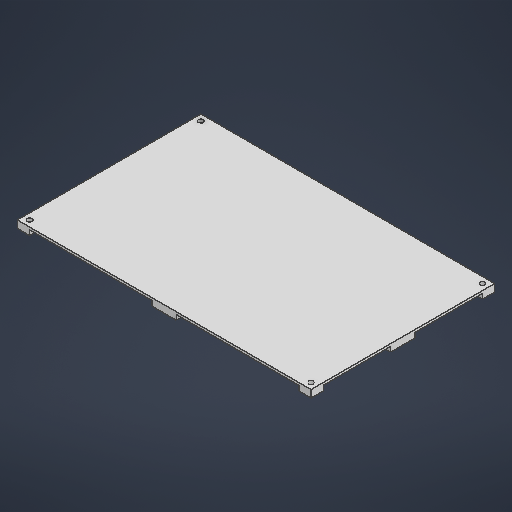
# Autodesk Inventor part: yellow_plate_cover
Saved by Autodesk Inventor 2026.1 (Build 301233000, 233)
## iProperties
Created: 2025-10-15
Part Number: yellow_plate_cover
Material: Generic
Document SubType Name: Modeling
Designer: emanuel
Density: 1 g/cm^3
Appearance: Default
Author: emanuel
Autodesk Inventor part; units mm, degrees
ref_plane "YZ Plane" through (0, 0, 0) normal (1, 0, 0) x (0, 1, 0)
ref_plane "XZ Plane" through (0, 0, 0) normal (0, 1, 0) x (-1, 0, 0)
ref_plane "XY Plane" through (0, 0, 0) normal (0, 0, 1) x (1, 0, 0)
sketch "Sketch1" plane through (0, 0, 0) normal (0, 1, 0) x (-1, 0, 0)
  line L0 (0, 0) -> (120, 0)
  line L1 (120, 0) -> (120, -75)
  line L2 (120, -75) -> (0, -75)
  line L3 (0, -75) -> (0, 0)
  line L4 (120, 0) -> (117.5, 0)
  line L5 (117.5, 0) -> (117.5, -2.5)
  line L6 (117.5, -2.5) -> (120, -2.5)
  line L7 (120, -2.5) -> (120, 0)
  line L8 (120, -75) -> (117.5, -75)
  line L9 (117.5, -75) -> (117.5, -72.5)
  line L10 (117.5, -72.5) -> (120, -72.5)
  line L11 (120, -72.5) -> (120, -75)
  line L12 (0, -75) -> (2.5, -75)
  line L13 (2.5, -75) -> (2.5, -72.5)
  line L14 (2.5, -72.5) -> (0, -72.5)
  line L15 (0, -72.5) -> (0, -75)
  line L16 (0, 0) -> (2.5, 0)
  line L17 (2.5, 0) -> (2.5, -2.5)
  line L18 (2.5, -2.5) -> (0, -2.5)
  line L19 (0, -2.5) -> (0, 0)
  line L20 (0, 0) -> (5, 0)
  line L21 (5, 0) -> (5, -5)
  line L22 (5, -5) -> (0, -5)
  line L23 (0, -5) -> (0, 0)
  line L24 (0, -75) -> (5, -75)
  line L25 (5, -75) -> (5, -70)
  line L26 (5, -70) -> (0, -70)
  line L27 (0, -70) -> (0, -75)
  line L28 (120, 0) -> (115, 0)
  line L29 (115, 0) -> (115, -5)
  line L30 (115, -5) -> (120, -5)
  line L31 (120, -5) -> (120, 0)
  line L32 (120, -75) -> (115, -75)
  line L33 (115, -75) -> (115, -70)
  line L34 (115, -70) -> (120, -70)
  line L35 (120, -70) -> (120, -75)
  circle A0 centre (117.5, -72.5) radius 1
  circle A1 centre (117.5, -2.5) radius 1
  circle A2 centre (2.5, -2.5) radius 1
  circle A3 centre (2.5, -72.5) radius 1
  line L36 (0, 0) -> (0, -37.5)
  line L37 (0, -37.5) -> (120, -37.5)
  line L38 (60, 0) -> (60, -75)
  line L39 (0, -32.5) -> (120, -32.5)
  line L40 (120, -32.5) -> (120, -42.5)
  line L41 (120, -42.5) -> (0, -42.5)
  line L42 (0, -42.5) -> (0, -32.5)
  line L43 (0, -32.5) -> (120, -42.5) construction
  line L44 (120, -32.5) -> (0, -42.5) construction
  line L45 (55, 0) -> (65, 0)
  line L46 (65, 0) -> (65, -75)
  line L47 (65, -75) -> (55, -75)
  line L48 (55, -75) -> (55, 0)
  line L49 (55, 0) -> (65, -75) construction
  line L50 (65, 0) -> (55, -75) construction
  point P0 (60, -37.5)
  point P1 (60, -37.5)
  point P2 (55, -32.5)
  point P3 (55, -42.5)
  point P4 (65, -42.5)
  point P5 (65, -32.5)
  dimension "d0" = 120
  dimension "d1" = 75
  dimension "d2" = 2.5
  dimension "d3" = 2.5
  dimension "d4" = 2.5
  dimension "d5" = 2.5
  dimension "d6" = 2.5
  dimension "d7" = 2.5
  dimension "d8" = 2.5
  dimension "d9" = 2.5
  dimension "d10" = 5
  dimension "d11" = 5
  dimension "d12" = 5
  dimension "d13" = 5
  dimension "d14" = 5
  dimension "d15" = 5
  dimension "d16" = 5
  dimension "d17" = 5
  dimension "d18" = 2
  dimension "d19" = 2
  dimension "d20" = 2
  dimension "d21" = 2
  dimension "d22" = 10
  dimension "d23" = 10
  constraints: 102 end point, 22 parallel, 11 horizontal, 11 perpendicular, 10 midpoint, 4 centre point, 4 coincident, 2 point on line
  measures "d0" distance of L1.end L2.end
  measures "d1" distance of L0.end L1.end
  measures "d2" distance of L6.end L5.end
  measures "d3" distance of L5.end L4.end
  measures "d4" distance of L9.end L10.end
  measures "d5" distance of L8.end L9.end
  measures "d6" distance of L14.end L13.end
  measures "d7" distance of L13.end L12.end
  measures "d8" distance of L17.end L18.end
  measures "d9" distance of L16.end L17.end
  measures "d10" distance of L21.end L22.end
  measures "d11" distance of L20.end L21.end
  measures "d12" distance of L26.end L25.end
  measures "d13" distance of L25.end L24.end
  measures "d14" distance of L30.end L29.end
  measures "d15" distance of L29.end L28.end
  measures "d16" distance of L33.end L34.end
  measures "d17" distance of L32.end L33.end
  measures "d18" diameter of A0
  measures "d19" diameter of A1
  measures "d20" diameter of A2
  measures "d21" diameter of A3
  measures "d22" distance of L39.end L40.end
  measures "d23" distance of L46.end L47.end
extrude "Extrusion1" add sketch "Sketch1" along normal blind 1 contours L0 L17 A2 L18 L3 | L0 L21 L22 L3 L18 A2 L17 | L0 L48 L39 L3 L22 L21 | L0 L38 L39 L48 | L39 L48 L37 L3 | L0 L46 L39 L38 | L39 L38 L37 L48 | L37 L48 L41 L3 | L0 L29 L30 L1 L39 L46 | L39 L46 L37 L38 | L37 L38 L41 L48 | L41 L48 L2 L25 L26 L3 | L0 L5 A1 L6 L1 L30 L29 | L39 L1 L37 L46 | L37 L46 L41 L38 | L41 L38 L2 L48 | L26 L25 L2 L13 A3 L14 L3 | L0 L1 L6 A1 L5 | L37 L1 L41 L46 | L41 L46 L2 L38 | L14 A3 L13 L2 L3 | L41 L1 L34 L33 L2 L46 | L1 L10 A0 L9 L2 L33 L34 | L1 L2 L9 A0 L10
extrude "Extrusion2" add sketch "Sketch1" against normal blind 2 contours L0 L17 A2 L18 L3 | L0 L21 L22 L3 L18 A2 L17 | L0 L38 L39 L48 | L39 L48 L37 L3 | L0 L46 L39 L38 | L39 L38 L37 L48 | L37 L48 L41 L3 | L39 L46 L37 L38 | L37 L38 L41 L48 | L0 L5 A1 L6 L1 L30 L29 | L39 L1 L37 L46 | L37 L46 L41 L38 | L41 L38 L2 L48 | L26 L25 L2 L13 A3 L14 L3 | L0 L1 L6 A1 L5 | L37 L1 L41 L46 | L41 L46 L2 L38 | L14 A3 L13 L2 L3 | L1 L10 A0 L9 L2 L33 L34 | L1 L2 L9 A0 L10
body "Solid1"
